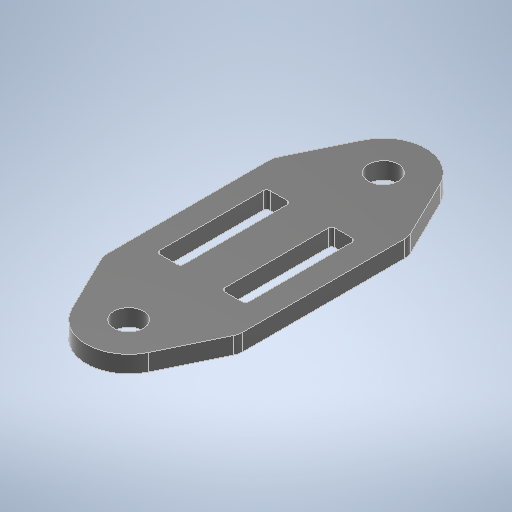
# Autodesk Inventor part: 3D_bno055_bottom
Saved by Autodesk Inventor 2025.1 (Build 291241020, 241B)
## iProperties
Created: 2024-08-31
Part Number: 3D_bno055_bottom
Material: 一般
Document SubType Name: Modeling
Designer: 8326d
Density: 1 g/cm^3
Appearance: 滑らか - 黒
Author: 8326d
## iProperties of the stored document 3D_bno055_bottom_3D プリント.ipt
Created: 2024-09-02
Part Number: 3D_bno055_bottom_3D プリント
Material: 一般
Document SubType Name: Modeling
Designer: 8326d
Density: 1 g/cm^3
Appearance: 既定
Author: 8326d
Autodesk Inventor part; units mm, degrees
ref_plane "YZ Plane" through (0, 0, 0) normal (1, 0, 0) x (0, 1, 0)
ref_plane "XZ Plane" through (0, 0, 0) normal (0, 1, 0) x (-1, 0, 0)
ref_plane "XY Plane" through (0, 0, 0) normal (0, 0, 1) x (1, 0, 0)
sketch "スケッチ1" plane through (0, 0, 0) normal (0, 1, 0) x (-1, 0, 0)
  line L0 (-8, 10) -> (8, 10)
  line L1 (8, 10) -> (8, -10)
  line L2 (8, -10) -> (-8, -10)
  line L3 (-8, -10) -> (-8, 10)
  line L4 (-8, 10) -> (8, -10) construction
  line L5 (8, 10) -> (-8, -10) construction
  circle A0 centre (0, 15) radius 5
  circle A1 centre (0, -15) radius 5
  line L6 (4.4944, 17.191) -> (8, 10)
  line L7 (-8, 10) -> (-4.4944, 17.191)
  line L8 (4.4944, -17.191) -> (8, -10)
  line L9 (-8, -10) -> (-4.4944, -17.191)
  point P0 (0, 0)
  dimension "d0" = 16
  dimension "d1" = 20
  dimension "d2" = 10
  dimension "d3" = 10
  constraints: 20 end point, 6 tangent, 4 point on circle, 2 centre point, 2 midpoint, 2 parallel, 2 vertical alignment, 1 horizontal, 1 perpendicular
  measures "d0" distance of L1.end L2.end
  measures "d1" distance of L0.end L1.end
  measures "d2" diameter of A0
  measures "d3" diameter of A1
extrude "押し出し1" add sketch "スケッチ1" along normal blind 2
sketch "スケッチ4" plane through (0, 2, 0) normal (0, 1, 0) x (1, 0, 0)
  arc A0 (-4.4944, -17.191) -> (4.4944, -17.191) centre (0, -15) ccw projected
  arc A1 (4.4944, 17.191) -> (-4.4944, 17.191) centre (0, 15) ccw projected
  point P0 (0, 0)
hole "穴1" at (0, 2, 15) at (0, 2, -15) direction (0, -1, 0) diameter 3.5 end through all
fillet "フィレット1" radius 2 4 edges at (8, 1, 10) (8, 1, -10) (-8, 1, -10) (-8, 1, 10)
sketch "スケッチ5" plane through (0, 2, 0) normal (0, 1, 0) x (1, 0, 0)
  line L0 (8, -9.5385) -> (8, 9.5385) projected
  line L1 (-8, -6.5) -> (8, -6.5)
  line L2 (8, -6.5) -> (8, 6.5)
  line L3 (8, 6.5) -> (-8, 6.5)
  line L4 (-8, 6.5) -> (-8, -6.5)
  line L5 (-8, -6.5) -> (8, 6.5) construction
  line L6 (8, -6.5) -> (-8, 6.5) construction
  line L7 (-2.4, -6.5) -> (2.4, -6.5)
  line L8 (2.4, -6.5) -> (2.4, 6.5)
  line L9 (2.4, 6.5) -> (-2.4, 6.5)
  line L10 (-2.4, 6.5) -> (-2.4, -6.5)
  line L11 (-2.4, -6.5) -> (2.4, 6.5) construction
  line L12 (2.4, -6.5) -> (-2.4, 6.5) construction
  line L13 (-8, 9.5385) -> (-8, -9.5385) projected
  line L14 (5.25, -6.5) -> (-5.25, -6.5)
  line L15 (-5.25, -6.5) -> (-5.25, 6.5)
  line L16 (-5.25, 6.5) -> (5.25, 6.5)
  line L17 (5.25, 6.5) -> (5.25, -6.5)
  line L18 (5.25, -6.5) -> (-5.25, 6.5) construction
  line L19 (-5.25, -6.5) -> (5.25, 6.5) construction
  point P0 (0, 0)
  dimension "d28" = 13
  dimension "d29" = 4.8
  dimension "d33" = 10.5
  constraints: 36 end point, 6 midpoint, 6 parallel, 3 horizontal, 3 perpendicular, 3 point on line
  measures "d28" distance of L3.end L1.start
  measures "d29" distance between parallel lines of L8 L10
  measures "d33" distance of L15.end L16.end
extrude "押し出し4" cut sketch "スケッチ5" against normal through all contours L1 L8 L3 L17 | L1 L15 L3 L10
fillet "フィレット2" radius 0.4 8 edges at (-2.4, 1, 6.5) (2.4, 1, 6.5) (2.4, 1, -6.5) (-2.4, 1, -6.5) (-5.25, 1, 6.5) (-5.25, 1, -6.5) (5.25, 1, -6.5) (5.25, 1, 6.5)
equation "\"d3\" = d2"
